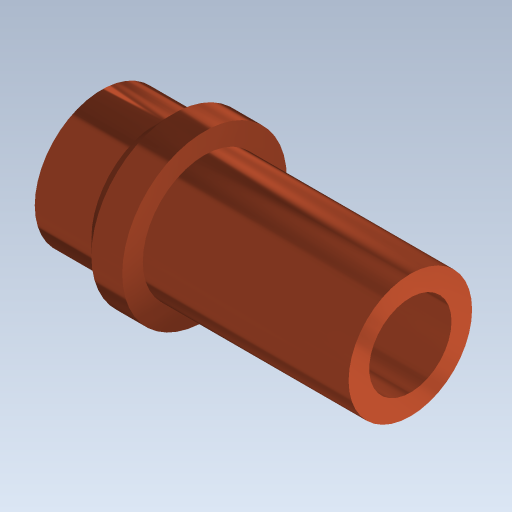
# Autodesk Inventor part: Pump-Motor-CW-Rotation:Pipe
Saved by Autodesk Inventor 2024.2 (Build 282272000, 272)
## iProperties
Created: 2025-06-16
Document SubType Name: Modeling
Density: 8.94 g/cm^3
Material: Copper
Mass: 20.8818 g
Surface Area: 22.1328 cm^2
Volume: 2.33577 cm^3
Appearance: Copper - Polished
Designer: cw
Author: cw
Autodesk Inventor part; units mm, degrees
ref_plane "YZ Plane" through (0, 0, 0) normal (1, 0, 0) x (0, 1, 0)
ref_plane "XZ Plane" through (0, 0, 0) normal (0, 1, 0) x (-1, 0, 0)
ref_plane "XY Plane" through (0, 0, 0) normal (0, 0, 1) x (1, 0, 0)
sketch "Sketch1" plane through (0, 0, 0) normal (0, 0, 1) x (1, 0, 0)
  line L0 (0, 0) -> (33.4625, 0)
  line L1 (0, 4) -> (0, 6.5)
  line L2 (0, 6.5) -> (5.5, 6.5)
  line L3 (5.5, 6.5) -> (7, 8)
  line L4 (7, 8) -> (10, 8)
  line L5 (10, 8) -> (10, 6)
  line L6 (10, 6) -> (30, 6)
  line L7 (30, 6) -> (30, 4)
  line L8 (30, 4) -> (0, 4)
  dimension "d1" = 8
  dimension "d2" = 13
  dimension "d3" = 5.5
  dimension "d4" = 135
  dimension "d5" = 16
  dimension "d6" = 3
  dimension "d7" = 12
  dimension "d8" = 30
  constraints: 18 end point, 5 parallel, 2 perpendicular, 1 horizontal, 1 vertical alignment
  measures "d1" diameter of L8 L0
  measures "d2" diameter of L2 L0
  measures "d3" distance of L1.end L2.end
  measures "d4" angle of L2 L3
  measures "d5" diameter of L4 L0
  measures "d6" distance of L3.end L4.end
  measures "d7" diameter of L6 L0
  measures "d8" distance of L7.end L1.start
revolve "Revolution1" add sketch "Sketch1" angle 360 about axis through (0, 0, 0) along (1, 0, 0)
body "Solid1"
